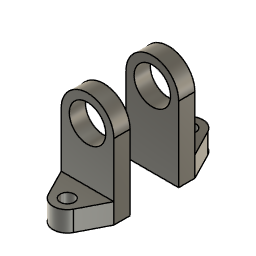
shaft_mount_rain (Autodesk Fusion 360 design; units mm, degrees)
Autodesk Fusion 360 part; units mm, degrees
sketch "Sketch1" plane through (0, 0, 0) normal (0, 0, 1) x (1, 0, 0)
  line L0 (6.5, 10) -> (-6.5, 10)
  line L1 (-6.5, 10) -> (-6.5, -10)
  line L2 (-6.5, -10) -> (6.5, -10)
  line L3 (6.5, -10) -> (6.5, 10)
  line L4 (6.5, 10) -> (-6.5, -10) construction
  line L5 (-6.5, 10) -> (6.5, -10) construction
  line L6 (-6.5, 10) -> (6.5, 10)
  line L7 (6.5, 10) -> (6.5, 6)
  line L8 (6.5, 6) -> (-6.5, 6)
  line L9 (-6.5, 6) -> (-6.5, 10)
  line L10 (-6.5, -10) -> (6.5, -10)
  line L11 (6.5, -10) -> (6.5, -6)
  line L12 (6.5, -6) -> (-6.5, -6)
  line L13 (-6.5, -6) -> (-6.5, -10)
  circle A0 centre (0, 15) radius 1.75
  circle A1 centre (0, -15) radius 1.75
  circle A2 centre (0, 15) radius 3.5
  circle A3 centre (0, -15) radius 3.5
  line L14 (-6.5, 10) -> (-3.1139, 16.598)
  line L15 (6.5, 10) -> (3.1139, 16.598)
  line L16 (-6.5, -10) -> (-3.1139, -16.598)
  line L17 (6.5, -10) -> (3.1139, -16.598)
  dimension "d1" = 13
  dimension "d2" = 20
  dimension "d3" = 4
  dimension "d4" = 4
  dimension "d5" = 3.5
  dimension "d6" = 15
  dimension "d7" = 3.5
  dimension "d8" = 15
  dimension "d9" = 7
  dimension "d10" = 7
  constraint horizontal L0
  constraint perpendicular L0 L1
  constraint parallel L0 L2
  constraint parallel L1 L3
  constraint coincident L4 origin
  constraint coincident L5 origin
  constraint horizontal L6
  constraint vertical L7
  constraint horizontal L8
  constraint vertical L9
  constraint coincident L3 L7.end
  constraint horizontal L10
  constraint vertical L11
  constraint horizontal L12
  constraint vertical L13
  constraint concentric A0 A2
  constraint concentric A1 A3
  constraint coincident A2 L14.end
  constraint tangent A2 L14
  constraint coincident A2 L15.end
  constraint tangent A2 L15
  constraint coincident A3 L16.end
  constraint tangent A3 L16
  constraint coincident A3 L17.end
  constraint tangent A3 L17
  constraint vertical origin A1.centre
  constraint vertical origin A0.centre
  measures "d1" distance of L1.end L2.end
  measures "d2" distance of L0.end L1.end
  measures "d3" distance of L0.end L8.end
  measures "d4" distance of L1.end L12.end
  measures "d5" diameter of A0
  measures "d6" distance of origin A0.centre
  measures "d7" diameter of A1
  measures "d8" distance of origin A1.centre
  measures "d9" diameter of A2
  measures "d10" diameter of A3
extrude "Extrude1" add sketch "Sketch1" along normal blind 5 contours L0 L1 L3 L6 L7 L8 L9 | L0 L6 A2 L14 L15 | A2 | L1 L2 L3 L10 L11 L12 L13 | L2 L10 A3 L16 L17 | A3 makes body 1 at (0.0436, 8.4183, 0) makes body 2 at (-0.0436, -8.4183, 0)
extrude "Extrude2" add sketch "Sketch1" along normal blind 25 contours L0 L1 L3 L6 L7 L8 L9 | L1 L2 L3 L10 L11 L12 L13 bodies 1 2
sketch "Sketch3" plane through (0, -10, 0) normal (0, -1, 0) x (1, 0, 0)
  line L0 (6.5, 5) -> (6.5, 25)
  line L1 (6.5, 25) -> (-6.5, 25)
  line L2 (-6.5, 25) -> (-6.5, 5)
  circle A0 centre (0, 18.5) radius 4.5
  circle A1 centre (0, 18.5) radius 6.5
  line L3 (-6.5, 5) -> (6.5, 5)
  dimension "d15" = 9
  dimension "d16" = 6.5
  constraint concentric A0 A1
  constraint tangent L0 A1
  measures "d15" diameter of A0
  measures "d16" distance of L1 A0.centre
extrude "Extrude4" cut sketch "Sketch3" against normal blind 20 contours L0 L1 A1 | L1 L2 A1 | A0 bodies 1 2
